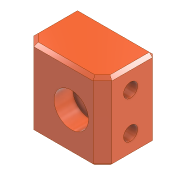
# Autodesk Inventor part: Print_Parts_R
Saved by Autodesk Inventor 2020.1 (Build 241239000, 239)
## iProperties
Created: 2020-10-05
Part Number: Print_Parts_R
Material: PC/ABS プラスチック
Document SubType Name: Modeling
Designer: kenta iguchi
Density: 0.357273 g/cm^3
Appearance: 滑らか - 淡いオレンジ
Author: kenta iguchi
Autodesk Inventor part; units mm, degrees
ref_plane "YZ Plane" through (0, 0, 0) normal (1, 0, 0) x (0, 1, 0)
ref_plane "XZ Plane" through (0, 0, 0) normal (0, 1, 0) x (-1, 0, 0)
ref_plane "XY Plane" through (0, 0, 0) normal (0, 0, 1) x (1, 0, 0)
sketch "スケッチ1" plane through (0, 0, 0) normal (0, 0, 1) x (1, 0, 0)
  circle A0 centre (0, 0) radius 5.1
  line L0 (10, -12.5) -> (-10, -12.5)
  line L1 (-10, -12.5) -> (-10, 12.5)
  line L2 (-10, 12.5) -> (10, 12.5)
  line L3 (10, 12.5) -> (10, -12.5)
  line L4 (10, -12.5) -> (-10, 12.5) construction
  line L5 (-10, -12.5) -> (10, 12.5) construction
  dimension "d0" = 10.2
  dimension "d1" = 25
  dimension "d2" = 20
  constraints: 12 end point, 2 midpoint, 2 parallel, 1 centre point, 1 coincident, 1 horizontal, 1 perpendicular
  measures "d0" diameter of A0
  measures "d1" distance of L0.end L1.end
  measures "d2" distance of L1.end L2.end
extrude "押し出し1" add sketch "スケッチ1" along normal blind 17
sketch "スケッチ2" plane through (0, 0, 17) normal (0, 0, 1) x (1, 0, 0)
  circle A0 centre (0, 0) radius 5.1 projected
extrude "押し出し2" add sketch "スケッチ2" against normal blind 12
sketch "スケッチ3" plane through (0, 0, 17) normal (0, 0, 1) x (1, 0, 0)
  point P0 (0, 0)
hole "穴1" at (0, 0, 17) direction (0, 0, -1) diameter 5.3 depth 58 counterbore diameter 11 counterbore depth 6
sketch "Sketch7" plane through (-10, -12.5, 0) normal (-1, 0, 0) x (0, 0, 1)
  line L0 (0, 25) -> (0, 0) projected
  line L1 (5, 7.4) -> (5, 17.6) projected
  line L2 (0, 17.6) -> (0, 7.4) projected
  point P0 (0, 12.5)
  point P1 (8, 6.5)
  point P2 (8, 18.5)
  dimension "d35" = 8
  dimension "d36" = 12
  dimension "d37" = 6
  constraints: 1 vertical alignment
  measures "d35" distance from line of L0 point (8, 6.5)
  measures "d36" distance of point (8, 6.5) point (8, 18.5)
  measures "d37" vertical distance of point (0, 12.5) point (8, 6.5)
hole "Hole3" at (-10, -6, 8) at (-10, 6, 8) direction (1, 0, 0) diameter 4.5 depth 58
chamfer "Chamfer2" distance 3 angle 45 1 edges at (10, 0, 17)
sketch "Sketch8" plane through (-10, -12.5, 0) normal (-1, 0, 0) x (0, 0, 1)
  circle A0 centre (8, 6.5) radius 2.25 projected
  circle A1 centre (8, 18.5) radius 2.25 projected
  line L0 (0, 25) -> (0, 0) projected
  line L1 (0, 0) -> (17, 0) projected
  line L2 (17, 25) -> (17, 0) projected
  line L3 (0, 25) -> (17, 25) projected
  point P0 (0, 12.5)
extrude "Extrusion5" add sketch "Sketch8" along normal blind 5
sketch "Sketch9" plane through (0, 0, 17) normal (0, 0, 1) x (1, 0, 0)
  line L0 (7, 12.5) -> (7, -12.5) projected
  line L1 (7, 12.5) -> (-15, 12.5) projected
  line L2 (-15, -12.5) -> (-15, 12.5) projected
  line L3 (7, -12.5) -> (-15, -12.5) projected
  circle A0 centre (0, 0) radius 5.5 projected
  line L4 (-15, 3.75) -> (-15, 8.25) projected
  line L5 (10, 8.25) -> (10, 3.75) projected
  line L6 (-15, -8.25) -> (-15, -3.75) projected
  line L7 (-15, -8.25) -> (-15, -3.75) projected
  line L8 (10, -3.75) -> (10, -8.25) projected
  line L9 (-10.9, 9.85) -> (-9.1, 9.85)
  line L10 (-9.1, 9.85) -> (-9.1, 2.15)
  line L11 (-9.1, 2.15) -> (-10.9, 2.15)
  line L12 (-10.9, 2.15) -> (-10.9, 9.85)
  line L13 (-10.9, 9.85) -> (-9.1, 2.15) construction
  line L14 (-9.1, 9.85) -> (-10.9, 2.15) construction
  line L15 (-10.9, -2.15) -> (-9.1, -2.15)
  line L16 (-9.1, -2.15) -> (-9.1, -9.85)
  line L17 (-9.1, -9.85) -> (-10.9, -9.85)
  line L18 (-10.9, -9.85) -> (-10.9, -2.15)
  line L19 (-10.9, -2.15) -> (-9.1, -9.85) construction
  line L20 (-9.1, -2.15) -> (-10.9, -9.85) construction
  line L21 (10, 8.25) -> (10, 3.75) projected
  point P0 (-10, 6)
  point P1 (-10, -6)
  point P2 (-10, 6)
  point P3 (-10, -6)
  point P4 (10, 6)
  point P5 (10, -6)
  point P6 (10, 6)
  dimension "d53" = 7.7
  dimension "d54" = 7.7
  dimension "d55" = 1.8
  dimension "d56" = 5
  constraints: 24 end point, 9 midpoint, 4 parallel, 2 horizontal, 2 horizontal alignment, 2 perpendicular, 2 vertical alignment
  measures "d53" distance of L11.end L9.start
  measures "d54" distance of L17.end L15.start
  measures "d55" distance of L16.end L17.end
  measures "d56" distance from line of point (-10, -6) L2
extrude "Extrusion6" cut sketch "Sketch9" against normal through all contours L9 L10 L11 L12 | L15 L16 L17 L18
sketch "Sketch10" plane through (0, 0, 17) normal (0, 0, 1) x (1, 0, 0)
  line L0 (-9.1, -2.15) -> (-9.1, -9.85) projected
  line L1 (-9.1, -9.85) -> (-10.9, -9.85) projected
  line L2 (-10.9, -9.85) -> (-10.9, -2.15) projected
  line L3 (-10.9, -2.15) -> (-9.1, -2.15) projected
  line L4 (-10.9, 9.85) -> (-9.1, 9.85) projected
  line L5 (-9.1, 9.85) -> (-9.1, 2.15) projected
  line L6 (-9.1, 2.15) -> (-10.9, 2.15) projected
  line L7 (-10.9, 2.15) -> (-10.9, 9.85) projected
  line L8 (7, 12.5) -> (7, -12.5) projected
  line L9 (7, 12.5) -> (-15, 12.5) projected
  line L10 (-15, -12.5) -> (-15, 12.5) projected
  line L11 (7, -12.5) -> (-15, -12.5) projected
  circle A0 centre (0, 0) radius 5.5 projected
extrude "Extrusion7" add sketch "Sketch10" against normal blind 5 contours L0 L1 L2 L3 | L4 L5 L6 L7
chamfer "Chamfer4" distance 3 angle 45 1 edges at (-15, 0, 17)
chamfer "面取り7" distance 1 angle 45 14 edges at (-15, 12.5, 7) (-13.5, 12.5, 15.5) (-2.5, 12.5, 17) (8.5, 12.5, 15.5) (10, 12.5, 7) (10, -12.5, 7) (8.5, -12.5, 15.5) (-2.5, -12.5, 17) (-13.5, -12.5, 15.5) (-15, -12.5, 7) (-2.5, 12.5, 0) (-2.5, -12.5, 0) (10, 0, 0) (-15, 0, 0)
sketch "スケッチ11" plane through (0, 0, 5) normal (0, 0, -1) x (-1, 0, 0)
  circle A0 centre (0, 0) radius 2.65 projected
  line L0 (2.65, 2.65) -> (-2.65, 2.65)
  line L1 (-2.65, 2.65) -> (-2.65, -2.65)
  line L2 (-2.65, -2.65) -> (2.65, -2.65)
  line L3 (2.65, -2.65) -> (2.65, 2.65)
  circle A1 centre (0, 0) radius 2.65 projected
  line L4 (2.65, 2.65) -> (-2.65, -2.65) construction
  line L5 (-2.65, 2.65) -> (2.65, -2.65) construction
  point P0 (2.65, 0)
  point P1 (0, -2.65)
  point P2 (0, 2.65)
  point P3 (-2.65, 0)
  constraints: 12 end point, 2 midpoint, 2 parallel, 2 tangent, 1 horizontal, 1 perpendicular
extrude "押し出し8" cut sketch "スケッチ11" against normal blind 0.6 contours L3 L2 A0 | A0 L0 L3 | A0 L1 L0 | L2 L1 A0
sketch "スケッチ12" plane through (0, 0, 5) normal (0, 0, -1) x (-1, 0, 0)
  line L0 (-2.65, 2.65) -> (2.65, 2.65) projected
  line L1 (2.65, -2.65) -> (-2.65, -2.65) projected
  circle A0 centre (0, 0) radius 5.1 projected
  line L2 (2.65, 5.3923) -> (-2.65, 5.3923)
  line L3 (-2.65, 5.3923) -> (-2.65, -5.3923)
  line L4 (-2.65, -5.3923) -> (2.65, -5.3923)
  line L5 (2.65, -5.3923) -> (2.65, 5.3923)
  line L6 (2.65, 5.3923) -> (-2.65, -5.3923) construction
  line L7 (-2.65, 5.3923) -> (2.65, -5.3923) construction
  point P0 (2.65, 2.65)
  point P1 (2.65, 4.3575)
  point P2 (-2.65, 4.3575)
  point P3 (2.65, -4.3575)
  point P4 (-2.65, -4.3575)
  constraints: 12 end point, 2 midpoint, 2 parallel, 1 horizontal, 1 perpendicular, 1 vertical alignment
extrude "押し出し9" cut sketch "スケッチ12" against normal blind 0.3 contours L3 A0 L5 L0 | L1 L5 A0 L3
equation "\"d37\" = 0.5 * d36"
